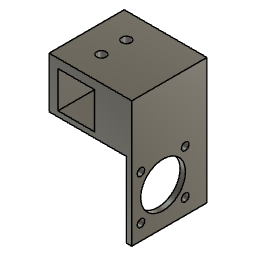
BG브라켓-R (Autodesk Fusion 360 design; units mm, degrees)
Autodesk Fusion 360 part; units mm, degrees
sketch "스케치1" plane through (0, 0, 0) normal (1, 0, 0) x (0, 1, 0)
  line L0 (21, 21) -> (-21, 21)
  line L1 (-21, 21) -> (-21, -21)
  line L2 (-21, -21) -> (21, -21)
  line L3 (21, -21) -> (21, 21)
  line L4 (21, 21) -> (-21, -21) construction
  line L5 (-21, 21) -> (21, -21) construction
  line L6 (-21, 0) -> (-3.5, 0)
  circle A0 centre (-3.5, 0) radius 17.5
  circle A1 centre (-3.5, 0) radius 12.5
  line L7 (-3.5, 0) -> (-15.8744, 12.3744)
  line L8 (-3.5, 0) -> (14, 0) construction
  circle A2 centre (-15.8744, 12.3744) radius 2.1
  circle A3 centre (-15.8744, -12.3744) radius 2.1
  circle A4 centre (8.8744, -12.3744) radius 2.1
  circle A5 centre (8.8744, 12.3744) radius 2.1
  line L9 (-21, 21) -> (21, 21)
  line L10 (21, 21) -> (21, 49.4)
  line L11 (21, 49.4) -> (-21, 49.4)
  line L12 (-21, 49.4) -> (-21, 21)
  dimension "d1" = 42
  dimension "d2" = 42
  dimension "d3" = 17.5
  dimension "d4" = 25
  dimension "d5" = 135
  dimension "d6" = 4.2
  dimension "d8" = 360
  dimension "d22" = 28.4
  constraint horizontal L0
  constraint perpendicular L0 L1
  constraint parallel L0 L2
  constraint parallel L1 L3
  constraint coincident L4 origin
  constraint coincident L5 origin
  constraint midpoint L1 L6.start
  constraint perpendicular L1 L6
  constraint coincident L6.end A0.centre
  constraint coincident L6.start A0
  constraint concentric A0 A1
  constraint horizontal L8
  constraint coincident A0 L7.end
  constraint coincident L7.end A2.centre
  constraint horizontal L9
  constraint vertical L10
  constraint horizontal L11
  constraint vertical L12
  measures "d1" distance of L1.end L2.end
  measures "d2" distance of L0.end L1.end
  measures "d3" distance of L6.start L6.end
  measures "d4" diameter of A1
  measures "d5" angle of L7 L8
  measures "d6" diameter of A2
  measures "d22" distance of L0.end L11.end
extrude "돌출1" add sketch "스케치1" along normal blind 3 contours L6 A0 A1 L7 A2 | L6 A0 A1 L7 A2 A3 A4 A5 | L0 L1 L2 L3 L9 | L0 L9 L10 L11 L12
extrude "돌출2" add sketch "스케치1" against normal blind 56 contours L0 L9 L10 L11 L12
sketch "스케치3" plane through (0, -21, 0) normal (0, -1, 0) x (1, 0, 0)
  line L0 (0, 21) -> (0, -21)
  line L1 (0, -21) -> (3, -21)
  line L2 (3, -21) -> (3, 49.4)
  line L3 (-56, 49.4) -> (-56, 21)
  line L4 (3, 49.4) -> (-56, 49.4)
  line L5 (-56, 21) -> (0, 21)
  line L6 (-56, 21) -> (-38.2, 21)
  line L7 (-38.2, 21) -> (-38.2, 24)
  line L8 (-38.2, 24) -> (-56, 24)
  line L9 (-56, 24) -> (-56, 21)
  line L10 (-38.2, 24) -> (-17.8, 24)
  line L11 (-17.8, 24) -> (-17.8, 44.4)
  line L12 (-17.8, 44.4) -> (-38.2, 44.4)
  line L13 (-38.2, 44.4) -> (-38.2, 24)
  dimension "d23" = 17.8
  dimension "d24" = 3
  dimension "d25" = 20.4
  dimension "d26" = 20.4
  constraint horizontal L6
  constraint vertical L7
  constraint horizontal L8
  constraint vertical L9
  constraint coincident L3.end L5.start
  constraint horizontal L10
  constraint vertical L11
  constraint horizontal L12
  constraint vertical L13
  measures "d23" distance of L3.end L6.end
  measures "d24" distance of L3.end L8.end
  measures "d25" distance of L7.end L10.end
  measures "d26" distance of L7.end L12.end
extrude "돌출3" cut sketch "스케치3" against normal blind 90 contours L10 L11 L12 L13
extrude "돌출4" cut 1 faces at (-56, 7, 39.9333) along direction (1, 0, 0) blind 12.8
sketch "스케치4" plane through (0, 0, 44.4) normal (0, 0, -1) x (1, 0, 0)
  line L0 (-38.2, -21) -> (-17.8, -21)
  line L1 (-17.8, -21) -> (-17.8, 21)
  line L2 (-17.8, 21) -> (-38.2, 21)
  line L3 (-38.2, 21) -> (-38.2, -21)
  line L4 (-28, 21) -> (-28, 7)
  circle A0 centre (-28, 7) radius 2.6
  line L5 (-28, 7) -> (-28, -7)
  circle A1 centre (-28, -7) radius 2.6
  dimension "d29" = 14
  dimension "d30" = 5.2
  dimension "d31" = 14
  dimension "d32" = 5.2
  constraint midpoint L2 L4.start
  constraint perpendicular L2 L4
  constraint coincident L4.end A0.centre
  constraint parallel L4 L5
  constraint coincident L5.end A1.centre
  measures "d29" distance of L4.start L4.end
  measures "d30" diameter of A0
  measures "d31" distance of L4.end L5.end
  measures "d32" diameter of A1
extrude "돌출5" cut sketch "스케치4" against normal blind 11 contours L4 A0 L5 | L4 A0 L5 | A1
sketch "스케치5" plane through (-38.2, 0, 0) normal (1, 0, 0) x (0, 1, 0)
  line L0 (21, 24) -> (21, 44.4)
  line L1 (21, 44.4) -> (-21, 44.4)
  line L2 (-21, 44.4) -> (-21, 24)
  line L3 (-21, 24) -> (21, 24)
  line L4 (-21, 34.2) -> (-7, 34.2)
  circle A0 centre (-7, 34.2) radius 2.6
  line L5 (-7, 34.2) -> (7, 34.2)
  circle A1 centre (7, 34.2) radius 2.6
  dimension "d35" = 14
  dimension "d36" = 5.2
  dimension "d37" = 14
  dimension "d38" = 5.2
  constraint midpoint L2 L4.start
  constraint perpendicular L2 L4
  constraint coincident L4.end A0.centre
  constraint parallel L4 L5
  constraint coincident L5.end A1.centre
  measures "d35" distance of L4.start L4.end
  measures "d36" diameter of A0
  measures "d37" distance of L4.end L5.end
  measures "d38" diameter of A1
extrude "돌출6" cut sketch "스케치5" against normal blind 11 contours L4 A0 L5 | L4 A0 L5 | A1
